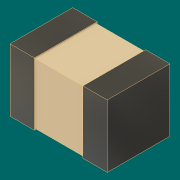
# Autodesk Inventor part: 0805 Capacitor
Saved by Autodesk Inventor 2016 (Build 200138000, 138)
## iProperties
Created: 2015-08-25
Part Number: 0805 Capacitor
Material: ABS Plastic
Document SubType Name: Modeling
Designer: Cosmic
Density: 1.06 g/cm^3
Appearance: Smooth - Off-White
Author: Cosmic
Autodesk Inventor part; units mm, degrees
ref_plane "YZ Plane" through (0, 0, 0) normal (1, 0, 0) x (0, 1, 0)
ref_plane "XZ Plane" through (0, 0, 0) normal (0, 1, 0) x (-1, 0, 0)
ref_plane "XY Plane" through (0, 0, 0) normal (0, 0, 1) x (1, 0, 0)
sketch "Sketch1" plane through (0, 0, 0) normal (0, 0, 1) x (1, 0, 0)
  line L0 (-1, -0.625) -> (1, -0.625)
  line L1 (1, -0.625) -> (1, 0.625)
  line L2 (1, 0.625) -> (-1, 0.625)
  line L3 (-1, 0.625) -> (-1, -0.625)
  line L4 (-1, -0.625) -> (1, 0.625) construction
  line L5 (1, -0.625) -> (-1, 0.625) construction
  point P0 (0, 0)
  dimension "d0" = 2
  dimension "d1" = 1.25
  constraints: 12 end point, 2 midpoint, 2 parallel, 1 horizontal, 1 perpendicular
  measures "d0" distance of L2.end L1.end
  measures "d1" distance of L1.end L0.end
extrude "Extrusion1" add sketch "Sketch1" along normal blind 1.25
sketch "Sketch2" plane through (1, -0.625, 0) normal (1, 0, 0) x (0, 0, -1)
  line L0 (0, 0) -> (0, 1.25) projected
  line L1 (0, 1.25) -> (-1.25, 1.25) projected
  line L2 (-1.25, 0) -> (-1.25, 1.25) projected
  line L3 (0, 0) -> (-1.25, 0) projected
  line L4 (-1.27, 1.27) -> (0.02, 1.27)
  line L5 (0.02, 1.27) -> (0.02, -0.02)
  line L6 (0.02, -0.02) -> (-1.27, -0.02)
  line L7 (-1.27, -0.02) -> (-1.27, 1.27)
  point P0 (0, 0.625)
  dimension "d4" = 0.02
  constraints: 8 end point, 3 other
  measures "d4" distance between parallel lines of L1 L4
extrude "Extrusion2" add sketch "Sketch2" against normal blind 0.5
sketch "Sketch3" plane through (-1, -0.625, 0) normal (-1, 0, 0) x (0, 0, 1)
  line L0 (0, 1.25) -> (0, 0) projected
  line L1 (0, 0) -> (1.25, 0) projected
  line L2 (1.25, 1.25) -> (1.25, 0) projected
  line L3 (0, 1.25) -> (1.25, 1.25) projected
  line L4 (1.27, -0.02) -> (-0.02, -0.02)
  line L5 (-0.02, -0.02) -> (-0.02, 1.27)
  line L6 (-0.02, 1.27) -> (1.27, 1.27)
  line L7 (1.27, 1.27) -> (1.27, -0.02)
  point P0 (0, 0.625)
  dimension "d7" = 0.02
  constraints: 8 end point, 3 other
  measures "d7" distance between parallel lines of L2 L7
extrude "Extrusion3" add sketch "Sketch3" against normal blind 0.5
body "Solid1"
